Autodesk Fusion 360 part; units mm, degrees
(part 2 of 2)
sketch "Esquisse3" plane through (0, 5, 0) normal (0, 1, 0) x (-1, 0, 0)
  line L0 (-85, 0) -> (-55, 0)
  circle A0 centre (-55, 5) radius 5
  line L1 (-55, 0) -> (-25, 0)
  line L2 (-25, 0) -> (-25, -5)
  line L3 (-25, -5) -> (-15, -5)
  line L4 (-15, -5) -> (-15, 0)
  line L5 (-15, 0) -> (0, 0)
  line L6 (0, 0) -> (0, 10)
  line L7 (0, 10) -> (-5, 10)
  line L8 (-5, 10) -> (-5, 20)
  line L9 (-5, 20) -> (-35, 20)
  line L10 (-35, 20) -> (-35, 10)
  line L11 (-35, 10) -> (-40, 10)
  line L12 (-40, 10) -> (-40, 20)
  line L13 (-40, 20) -> (-70, 20)
  line L14 (-70, 20) -> (-70, 10)
  line L15 (-70, 10) -> (-75, 10)
  line L16 (-75, 10) -> (-75, 20)
  line L17 (-75, 20) -> (-105, 20)
  line L18 (-105, 20) -> (-105, 10)
  line L19 (-105, 10) -> (-110, 10)
  line L20 (-110, 10) -> (-110, 20)
  line L21 (-110, 20) -> (-140, 20)
  line L22 (-140, 20) -> (-140, 10)
  line L23 (-140, 10) -> (-145, 10)
  line L24 (-145, 10) -> (-145, 20)
  line L25 (-145, 20) -> (-175, 20)
  line L26 (-175, 20) -> (-175, 10)
  line L27 (-175, 10) -> (-180, 10)
  line L28 (-180, 10) -> (-180, 20)
  line L29 (-180, 20) -> (-210, 20)
  line L30 (-210, 20) -> (-210, 10)
  line L31 (-210, 10) -> (-215, 10)
  line L32 (-215, 10) -> (-215, 20)
  line L33 (-215, 20) -> (-245, 20)
  line L34 (-245, 20) -> (-245, 10)
  line L35 (-245, 10) -> (-250, 10)
  line L36 (-250, 10) -> (-250, 20)
  line L37 (-250, 20) -> (-280, 20)
  line L38 (-280, 20) -> (-280, 10)
  line L39 (-280, 10) -> (-285, 10)
  line L40 (-285, 10) -> (-285, 0)
  line L41 (-285, 0) -> (-265, 0)
  circle A1 centre (-265, 5) radius 5
  line L42 (-265, 0) -> (-235, 0)
  line L43 (-235, 0) -> (-235, -5)
  line L44 (-235, -5) -> (-225, -5)
  line L45 (-225, -5) -> (-225, 0)
  line L46 (-225, 0) -> (-195, 0)
  circle A2 centre (-195, 5) radius 5
  line L47 (-195, 0) -> (-165, 0)
  line L48 (-165, 0) -> (-165, -5)
  line L49 (-165, -5) -> (-155, -5)
  line L50 (-155, -5) -> (-155, 0)
  line L51 (-155, 0) -> (-125, 0)
  circle A3 centre (-125, 5) radius 5
  line L52 (-125, 0) -> (-95, 0)
  line L53 (-95, 0) -> (-95, -5)
  line L54 (-95, -5) -> (-85, -5)
  line L55 (-85, -5) -> (-85, 0)
  circle A4 centre (-230, 5) radius 5
  circle A5 centre (-20, 5) radius 5
  circle A6 centre (-160, 5) radius 5
  circle A7 centre (-90, 5) radius 5
